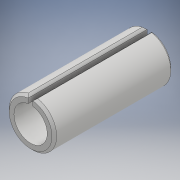
# Autodesk Inventor part: M2x5彈簧銷
Saved by Autodesk Inventor 2018 (Build 220112000, 112)
## iProperties
Created: 2025-06-12
Part Number: M2x5彈簧銷
Material: 一般
Document SubType Name: Modeling
Designer: User
Density: 1 g/cm^3
Appearance: 預設
Author: User
Autodesk Inventor part; units mm, degrees
ref_plane "YZ Plane" through (0, 0, 0) normal (1, 0, 0) x (0, 1, 0)
ref_plane "XZ Plane" through (0, 0, 0) normal (0, 1, 0) x (-1, 0, 0)
ref_plane "XY Plane" through (0, 0, 0) normal (0, 0, 1) x (1, 0, 0)
sketch "草圖1" plane through (0, 0, 0) normal (0, 1, 0) x (-1, 0, 0)
  circle A0 centre (0, 0) radius 1
  circle A1 centre (0, 0) radius 0.7
  dimension "d0" = 2
  dimension "d1" = 1.4
  constraints: 2 centre point, 2 coincident
  measures "d0" diameter of A0
  measures "d1" diameter of A1
extrude "擠出1" add sketch "草圖1" along normal blind 5
sketch "草圖2" plane through (0, 0, 0) normal (0, -1, 0) x (1, 0, 0)
  line L0 (-0.1, 1.1657) -> (0.1, 1.1657)
  line L1 (0.1, 1.1657) -> (0.1, 0.5445)
  line L2 (0.1, 0.5445) -> (-0.1, 0.5445)
  line L3 (-0.1, 0.5445) -> (-0.1, 1.1657)
  point P0 (0, 0)
  dimension "d4" = 0.1
  dimension "d5" = 0.2
  constraints: 8 end point, 2 parallel, 1 horizontal, 1 perpendicular
  measures "d4" distance from line of point (0, 0) L1
  measures "d5" distance between parallel lines of L1 L3
extrude "擠出2" cut sketch "草圖2" against normal blind 5
chamfer "倒角1" distance 0.1 angle 45 2 edges at (-0.1, 2.5, 0.995) (0.1, 2.5, 0.995)
chamfer "倒角2" distance 0.1 angle 45 2 edges at (0, 0, -1) (0, 5, -1)
